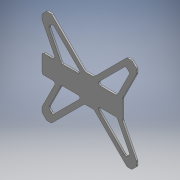
# Autodesk Inventor part: FR4
Saved by Autodesk Inventor 2016 (Build 200138000, 138)
## iProperties
Created: 2018-05-21
Part Number: FR4
Material: Generic
Document SubType Name: Modeling
Designer: suku
Density: 1 g/cm^3
Appearance: Default
Author: suku
Autodesk Inventor part; units mm, degrees
ref_plane "YZ Plane" through (0, 0, 0) normal (1, 0, 0) x (0, 1, 0)
ref_plane "XZ Plane" through (0, 0, 0) normal (0, 1, 0) x (-1, 0, 0)
ref_plane "XY Plane" through (0, 0, 0) normal (0, 0, 1) x (1, 0, 0)
sketch "Sketch1" plane through (0, 0, 0) normal (0, 1, 0) x (-1, 0, 0)
  line L0 (50, 45) -> (50, 40)
  line L1 (50, 40) -> (35, 10)
  line L2 (45, 50) -> (40, 50)
  line L3 (-45, 50) -> (-40, 50)
  line L4 (-50, 45) -> (-50, 40)
  line L5 (-50, 40) -> (-35, 10)
  line L6 (50, 10) -> (50, 0)
  line L7 (-35, 10) -> (-35, 0)
  line L8 (-40, 50) -> (-5, 15)
  line L9 (5, 15) -> (40, 50)
  line L10 (35, 10) -> (50, 10)
  line L11 (5, 15) -> (-5, 15)
  line L12 (-35, 0) -> (50, 0)
  line L13 (7.0711, 10) -> (29.4098, 10)
  line L14 (-29.4098, 10) -> (-7.0711, 10)
  line L15 (-29.4098, 10) -> (-43.0069, 37.1941)
  line L16 (43.0069, 37.1941) -> (29.4098, 10)
  line L17 (38.636, 41.565) -> (7.0711, 10)
  line L18 (43.0069, 37.1941) -> (38.636, 41.565)
  line L19 (-43.0069, 37.1941) -> (-38.636, 41.565)
  line L20 (-38.636, 41.565) -> (-7.0711, 10)
  line L21 (45, 50) -> (50, 45)
  line L22 (-45, 50) -> (-50, 45)
  point P0 (0, 0)
  point P1 (-50, 50)
  point P2 (50, 50)
  dimension "d6" = 10
  dimension "d7" = 10
  dimension "d8" = 10
  dimension "d9" = 15
  dimension "d10" = 100
  dimension "d20" = 14
  dimension "d21" = 5
  dimension "d22" = 5
  dimension "d23" = 10
  dimension "d25" = 5
  dimension "d26" = 14
  dimension "d27" = 10
  dimension "d28" = 5
  dimension "d29" = 5
  dimension "d30" = 5
  dimension "d31" = 5
  constraints: 46 end point, 5 horizontal, 4 point on line, 3 parallel, 2 collinear, 1 vertical
  measures "d6" distance of point (50, 50) L2.end
  measures "d7" distance of point (-50, 50) L3.end
  measures "d8" distance of point (-50, 50) L4.end
  measures "d9" distance of L6.start L1.end
  measures "d10" distance between parallel lines of L0 L4
  measures "d20" distance from line of point (50, 50) L18
  measures "d21" distance between parallel lines of L9 L17
  measures "d22" distance between parallel lines of L1 L16
  measures "d23" distance between parallel lines of L10 L12
  measures "d25" distance between parallel lines of L5 L15
  measures "d26" distance from line of point (-50, 50) L19
  measures "d27" distance of point (50, 50) L0.end
  measures "d28" distance of L2.start point (50, 50)
  measures "d29" distance of L0.start point (50, 50)
  measures "d30" distance of L3.start point (-50, 50)
  measures "d31" distance of L4.start point (-50, 50)
extrude "Extrusion1" add sketch "Sketch1" along normal blind 1.6
fillet "Fillet1" radius 2 21 edges at (-29.4098, 0.8, 10) (-7.0711, 0.8, 10) (7.0711, 0.8, 10) (-5, 0.8, 15) (5, 0.8, 15) (43.0069, 0.8, 37.1941) (35, 0.8, 10) (29.4098, 0.8, 10) (-35, 0.8, 10) (-50, 0.8, 10) (-50, 0.8, 40) (-40, 0.8, 50) (40, 0.8, 50) (50, 0.8, 40) (-45, 0.8, 50) (-50, 0.8, 45) (-43.0069, 0.8, 37.1941) (-38.636, 0.8, 41.565) (38.636, 0.8, 41.565) (45, 0.8, 50) (50, 0.8, 45)
mirror "Mirror1" about plane through (35, 0, 0) normal (0, 0, -1) of "Extrusion1", "Fillet1"
equation "\"d29\" = d28"
equation "\"d30\" = d28"
equation "\"d31\" = d30"
body "Solid1"
